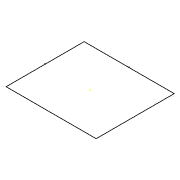
# Autodesk Inventor part: Lower Rod Fulcrum
Saved by Autodesk Inventor 2015 (Build 190159000, 159)
## iProperties
Created: 2020-04-22
Part Number: Lower Rod Fulcrum
Material: Generic
Document SubType Name: Modeling
Designer: Ghassan Yusuf
Density: 1 g/cm^3
Appearance: Default
Author: Ghassan Yusuf
Autodesk Inventor part; units mm, degrees
ref_plane "YZ Plane" through (0, 0, 0) normal (1, 0, 0) x (0, 1, 0)
ref_plane "XZ Plane" through (0, 0, 0) normal (0, 1, 0) x (-1, 0, 0)
ref_plane "XY Plane" through (0, 0, 0) normal (0, 0, 1) x (1, 0, 0)
sketch "Sketch1" plane through (0, 0, 0) normal (0, 0, 1) x (1, 0, 0)
  line L0 (-30.15, 25) -> (30.15, 25)
  line L1 (30.15, 25) -> (30.15, -25)
  line L2 (30.15, -25) -> (-30.15, -25)
  line L3 (-30.15, -25) -> (-30.15, 25)
  line L4 (-30.15, 25) -> (-25.15, 25)
  line L5 (-25.15, 25) -> (-25.15, -25)
  line L6 (-25.15, -25) -> (-30.15, -25)
  line L7 (-30.15, -25) -> (-30.15, 25)
  line L8 (30.15, 25) -> (25.15, 25)
  line L9 (25.15, 25) -> (25.15, -25)
  line L10 (25.15, -25) -> (30.15, -25)
  line L11 (30.15, -25) -> (30.15, 25)
  point P0 (0, 0)
  point P1 (-30.15, 0)
  point P2 (0, 25)
  dimension "d0" = 60.3
  dimension "d1" = 50
  dimension "d2" = 5
  dimension "d3" = 5
  constraints: 24 end point, 6 parallel, 3 horizontal, 3 perpendicular, 2 midpoint, 2 point on line, 1 horizontal alignment, 1 vertical alignment
  measures "d0" distance of L0.start L0.end
  measures "d1" distance of L2.end L0.start
  measures "d2" distance of L5.end L6.end
  measures "d3" distance between parallel lines of L1 L9
extrude "Extrusion1" add sketch "Sketch1" along normal blind 18 contours L0 L5 L2 L3 | L0 L1 L2 L9
sketch "Sketch2" plane through (0, 0, 18) normal (0, 0, 1) x (1, 0, 0)
  line L0 (-30.15, 25) -> (30.15, 25)
  line L1 (30.15, 25) -> (30.15, -25)
  line L2 (30.15, -25) -> (-30.15, -25)
  line L3 (-30.15, -25) -> (-30.15, 25)
  point P0 (0, 0)
  constraints: 8 end point, 2 parallel, 1 horizontal, 1 perpendicular
extrude "Extrusion2" add sketch "Sketch2" along normal blind 5
body "Solid1"
